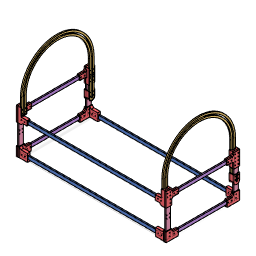
Locolus V2.1 (with correction) v3 (Autodesk Fusion 360 design; units mm, degrees)
Autodesk Fusion 360 part; units mm, degrees
note: some values were not read from the file. Chosen so that the rebuilt part matches the saved one: which bodies a step acts on; which face or edge a step refers to. Set by a fixed rule: which sketch regions a step uses.
sketch "Sketch1" plane through (0, 0, 0) normal (1, 0, 0) x (0, 0, -1) in component "Door"
  line L0 (0, 0) -> (0, 50)
  arc A0 (200, 50) -> (0, 50) centre (100, 50) ccw
  line L1 (200, 50) -> (200, 0)
  line L2 (-5, 0) -> (-5, 50)
  arc A1 (205, 50) -> (-5, 50) centre (100, 50) ccw
  line L3 (205, 50) -> (205, 0)
  line L4 (-9, 0) -> (-9, 50)
  arc A2 (209, 50) -> (-9, 50) centre (100, 50) ccw
  line L5 (209, 50) -> (209, 0)
  line L6 (-14, 0) -> (-14, 50)
  arc A3 (214, 50) -> (-14, 50) centre (100, 50) ccw
  line L7 (214, 50) -> (214, 0)
  line L8 (-5, 0) -> (0, 0)
  line L9 (200, 0) -> (205, 0)
  line L10 (209, 0) -> (214, 0)
  line L11 (-14, 0) -> (-9, 0)
  line L12 (-11.5, 0) -> (-11.5, 50) construction
  line L13 (-2.5, 0) -> (-2.5, 50) construction
  circle A4 centre (-2.5, 5) radius 1.4
  circle A5 centre (-2.5, 15) radius 1.4
  line L14 (-7, 0) -> (-7, 19) construction
  circle A6 centre (-11.5, 5) radius 1.4
  circle A7 centre (-11.5, 15) radius 1.4
  line L15 (100, 50) -> (100, 0) construction
  circle A8 centre (211.5, 15) radius 1.4
  circle A9 centre (211.5, 5) radius 1.4
  circle A10 centre (202.5, 5) radius 1.4
  circle A11 centre (202.5, 15) radius 1.4
  line L16 (200, 0) -> (205, 0)
  line L17 (205, 0) -> (205, -60)
  line L18 (200, -60) -> (200, 0)
  line L19 (209, 0) -> (214, 0)
  line L20 (214, 0) -> (214, -60)
  line L21 (209, -60) -> (209, 0)
  circle A12 centre (202.5, -5) radius 1.4
  circle A13 centre (211.5, -15) radius 1.4
  circle A14 centre (202.5, -15) radius 1.4
  circle A15 centre (211.5, -5) radius 1.4
  line L22 (207, -60) -> (207, -43) construction
  line L23 (211.5, -60) -> (211.5, -39) construction
  line L24 (202.5, -60) -> (202.5, -39) construction
  circle A16 centre (211.5, -55) radius 1.4
  circle A17 centre (211.5, -45) radius 1.4
  circle A18 centre (202.5, -55) radius 1.4
  circle A19 centre (202.5, -45) radius 1.4
  arc A20 (205, -60) -> (209, -60) centre (207, -60) ccw
  arc A21 (200, -60) -> (214, -60) centre (207, -60) ccw
  point P0 (202.5, -45)
  dimension "d1" = 100
  dimension "d2" = 50
  dimension "d3" = -5
  dimension "d4" = -9
  dimension "d5" = -14
  dimension "d6" = 50
  dimension "d7" = 2.8
  dimension "d8" = 5
  dimension "d9" = 2.8
  dimension "d10" = 15
  dimension "d11" = 2
  dimension "d14" = 5
  dimension "d15" = 60
  dimension "d16" = 5
  dimension "d17" = 60
  dimension "d38" = 2
  dimension "d39" = 2.8
  dimension "d40" = 2.8
  dimension "d50" = 5
  dimension "d51" = 9
  dimension "d52" = 15
  constraint coincident L0.start L8.end
  constraint vertical L0
  constraint tangent L0 A0
  constraint tangent A0 L1
  constraint vertical L1
  constraint perpendicular L0 L8
  constraint perpendicular L7 L10
  constraint perpendicular L4 L11
  constraint midpoint L11 L12.start
  constraint perpendicular L11 L12
  constraint midpoint L8 L13.start
  constraint perpendicular L8 L13
  constraint coincident L13 A4.centre
  constraint coincident L13 A5.centre
  constraint parallel L2 L14
  constraint symmetric A4 L14 A6
  constraint symmetric A5 L14 A7
  constraint coincident A0.centre A1.centre
  constraint vertical L15
  constraint symmetric A4 L15 A10
  constraint symmetric A5 L15 A11
  constraint symmetric A6 L15 A9
  constraint symmetric A7 L15 A8
  constraint horizontal L16
  constraint vertical L17
  constraint vertical L18
  constraint horizontal L19
  constraint vertical L20
  constraint vertical L21
  constraint symmetric L9 A8 A13
  constraint symmetric L9 A9 A15
  constraint symmetric L9 A10 A12
  constraint symmetric L9 A11 A14
  constraint coincident L23 A16.centre
  constraint coincident L23 A17.centre
  constraint symmetric L22 A16 A18
  constraint symmetric L22 A17.centre P0
  constraint symmetric L22 A17 A19
  constraint tangent L17 A20
  constraint tangent L21 A20
  constraint tangent L18 A21
  constraint tangent L20 A21
  constraint vertical L23
  constraint vertical L24
  measures "d1" radius of A0
  measures "d2" distance of L0.start L0.end
  measures "d6" distance of A0.start L1.end
  measures "d7" diameter of A4
  measures "d8" distance of L8 A4.centre
  measures "d9" diameter of A5
  measures "d10" distance of L8 A5.centre
  measures "d11" distance of L4 L14
  measures "d14" distance of L1.end L3.end
  measures "d15" distance of L1.end L18.start
  measures "d16" distance of L5.end L7.end
  measures "d17" distance of L5.end L21.start
  measures "d38" distance of L17 L22
  measures "d39" diameter of A16
  measures "d40" diameter of A17
  measures "d50" vertical distance of A18.centre L22.start
  measures "d51" distance of A16.centre A18.centre
  measures "d52" vertical distance of P0 L22.start
extrude "Extrude1" add sketch "Sketch1" against normal blind 4 contours L0 A0 L1 L2 A1 L3 L8 L9 L16 | L4 A2 L5 L6 A3 L7 L10 L11 L19 makes body 1 at (0, 38.8, 11.5) makes body 2 at (0, 38.798, 2.4569) in component "Door"
extrude "Extrude2" add sketch "Sketch1" against normal blind 4 separate body contours L9 L10 L16 L17 L18 L19 L20 L21 A20 A21 makes body 3 in component "Door"
sketch "Sketch1 (2)" plane through (0, 0, 0) normal (1, 0, 0) x (0, 0, -1) in component "Transverse carcas"
  line L0 (195, 0) -> (5, 0)
  line L1 (5, 0) -> (5, 10)
  line L2 (5, 10) -> (195, 10)
  line L3 (195, 10) -> (195, 0)
  line L4 (200, 50) -> (200, 0)
  line L5 (0, 0) -> (0, 50)
  circle A0 centre (190, 5) radius 1.4
  circle A1 centre (180, 5) radius 1.4
  line L6 (100, 10) -> (100, 0) construction
  line L7 (100, 50) -> (100, 0) construction
  circle A2 centre (20, 5) radius 1.4
  circle A3 centre (10, 5) radius 1.4
  circle A4 centre (190, 5) radius 5
  circle A5 centre (10, 5) radius 5
  line L8 (195, -110) -> (5, -110)
  line L9 (5, -110) -> (5, -100)
  line L10 (5, -100) -> (195, -100)
  line L11 (195, -100) -> (195, -110)
  line L12 (200, -60) -> (200, 0)
  line L13 (195, -50) -> (5, -50) construction
  circle A6 centre (190, -105) radius 1.4
  circle A7 centre (190, -105) radius 5
  circle A8 centre (180, -105) radius 1.4
  circle A9 centre (20, -105) radius 1.4
  circle A10 centre (10, -105) radius 5
  circle A11 centre (10, -105) radius 1.4
  point P0 (100, 50)
  dimension "d20" = 5
  dimension "d21" = 5
  dimension "d22" = 10
  dimension "d23" = 40
  dimension "d24" = 2.8
  dimension "d25" = 5
  dimension "d26" = 2.8
  dimension "d27" = 15
  dimension "d28" = 5
  dimension "d29" = 5
  dimension "d30" = 100
  dimension "d31" = 10
  dimension "d32" = 5
  dimension "d33" = 5
  dimension "d34" = 50
  constraint horizontal L0
  constraint vertical L1
  constraint horizontal L2
  constraint vertical L3
  constraint midpoint L2 L6.start
  constraint midpoint L0 L6.end
  constraint symmetric A0 L7 A3
  constraint symmetric A1 L7 A2
  constraint concentric A0 A4
  constraint tangent L0 A4
  constraint concentric A3 A5
  constraint tangent L0 A5
  constraint horizontal L8
  constraint vertical L9
  constraint horizontal L10
  constraint vertical L11
  constraint parallel L0 L13
  constraint symmetric A0 L13 A6
  constraint symmetric A1 L13 A8
  constraint symmetric A2 L13 A9
  constraint symmetric A3 L13 A11
  constraint symmetric A4 L13 A7
  constraint symmetric A5 L13 A10
  measures "d20" distance of L3 L4
  measures "d21" distance of L1 L5
  measures "d22" distance of L0.start L2.end
  measures "d23" distance of L2 P0
  measures "d24" diameter of A0
  measures "d25" distance of L3 A0.centre
  measures "d26" diameter of A1
  measures "d27" distance of L3 A1.centre
  measures "d28" distance of L2 A0.centre
  measures "d29" distance of L2 A1.centre
  measures "d30" distance of L0 L10
  measures "d31" distance of L8 L10
  measures "d32" distance of L11 L12
  measures "d33" distance of L5 L9
  measures "d34" distance of L0 L13
extrude "Extrude1'" add sketch "Sketch1 (2)" against normal blind 4 from surface at -9 separate body contours L0 L2 A4 A5 | A4 | A5 | L8 L10 A7 A10 | A7 | A10 makes body 4 at (-9, 1.2159, -73.4541) makes body 5 at (-9, -108.7841, -73.4541) in component "Transverse carcas"
sketch "Sketch1 (3)" plane through (0, 0, 0) normal (1, 0, 0) x (0, 0, -1) in component "High carcas"
  line L0 (214, 20) -> (200, 20)
  line L1 (200, 20) -> (200, -110)
  line L2 (200, -110) -> (214, -110)
  line L3 (214, -110) -> (214, 20)
  line L4 (214, 0) -> (214, -60)
  line L5 (200, -60) -> (200, 0)
  line L6 (190, -110) -> (10, -110)
  circle A0 centre (211.5, 15) radius 1.4
  circle A1 centre (202.5, 15) radius 1.4
  circle A2 centre (211.5, -15) radius 1.4
  circle A3 centre (211.5, -5) radius 1.4
  circle A4 centre (211.5, 5) radius 1.4
  circle A5 centre (202.5, 5) radius 1.4
  circle A6 centre (202.5, -5) radius 1.4
  circle A7 centre (202.5, -15) radius 1.4
  circle A8 centre (202.5, -55) radius 1.4
  line L7 (202.5, -60) -> (202.5, -39)
  circle A9 centre (202.5, -45) radius 1.4
  circle A10 centre (211.5, -55) radius 1.4
  circle A11 centre (211.5, -45) radius 1.4
  line L8 (214, 50) -> (214, 0)
  line L9 (100, 50) -> (100, 0)
  circle A12 centre (-11.5, 15) radius 1.4
  circle A13 centre (-2.5, -55) radius 1.4
  line L10 (0, -60) -> (0, 0)
  line L11 (0, -110) -> (-14, -110)
  circle A14 centre (-11.5, -45) radius 1.4
  circle A15 centre (-11.5, -55) radius 1.4
  circle A16 centre (-2.5, -45) radius 1.4
  line L12 (-2.5, -60) -> (-2.5, -39)
  line L13 (-14, -110) -> (-14, 20)
  line L14 (0, 20) -> (0, -110)
  line L15 (-14, 0) -> (-14, -60)
  circle A17 centre (-11.5, 5) radius 1.4
  circle A18 centre (-2.5, 15) radius 1.4
  circle A19 centre (-2.5, 5) radius 1.4
  circle A20 centre (-2.5, -15) radius 1.4
  circle A21 centre (-2.5, -5) radius 1.4
  line L16 (-14, 20) -> (0, 20)
  line L17 (214, -110) -> (235.1047, -110) construction
  line L18 (205, -110) -> (205, -95) construction
  circle A22 centre (205, -105) radius 1.4
  circle A23 centre (205, -95) radius 1.4
  circle A24 centre (-5, -105) radius 1.4
  circle A25 centre (-5, -95) radius 1.4
  line L19 (-5, -110) -> (-5, -95) construction
  point P0 (211.5, 15)
  point P1 (211.5, -15)
  point P2 (-11.5, -15)
  point P3 (-14, 0)
  point P4 (-11.5, 15)
  dimension "d44" = 5
  dimension "d104" = 5
  dimension "d105" = 2.8
  dimension "d106" = 2.8
  dimension "d107" = 5
  dimension "d108" = 15
  constraint horizontal L0
  constraint vertical L1
  constraint horizontal L2
  constraint vertical L3
  constraint collinear L3 L4
  constraint collinear L1 L5
  constraint collinear L2 L6
  constraint symmetric L0.start L9 L13.end
  constraint symmetric L0.end L9 L14.start
  constraint symmetric L1.end L9 L11.start
  constraint symmetric L2.end L9 L11.end
  constraint symmetric L4.start L9 P3
  constraint symmetric L4.end L9 L15.end
  constraint symmetric L5.start L9 L10.start
  constraint symmetric L5.end L9 L10.end
  constraint symmetric P0 L9 P4
  constraint symmetric A0 L9 A12
  constraint symmetric A1 L9 A18
  constraint symmetric P1 L9 P2
  constraint symmetric A4 L9 A17
  constraint symmetric A5 L9 A19
  constraint symmetric A6 L9 A21
  constraint symmetric A7 L9 A20
  constraint symmetric A8 L9 A13
  constraint symmetric L7.start L9 L12.start
  constraint symmetric L7.end L9 L12.end
  constraint symmetric A9 L9 A16
  constraint symmetric A10 L9 A15
  constraint symmetric A11 L9 A14
  constraint horizontal L17
  constraint coincident L2 L18.start
  constraint perpendicular L2 L18
  constraint coincident L18 A22.centre
  constraint coincident L18 A23.centre
  constraint symmetric L9 L18.start L19.start
  constraint symmetric L9 L18.end A25.centre
  constraint symmetric L9 A22 A24
  constraint symmetric L9 A23 A25
  measures "d44" distance of L0 P0
  measures "d104" distance of L1 L18
  measures "d105" diameter of A22
  measures "d106" diameter of A23
  measures "d107" distance of L2 A22.centre
  measures "d108" distance of L2 L18.end
extrude "Extrude1''" add sketch "Sketch1 (3)" along normal blind 4 from surface at -13 separate body makes body 6 at (-13, -18.4191, 9.6485) makes body 7 at (-13, -68.7664, -206.3764) in component "High carcas"
ref_plane "WorkPlane1" through (-11, -45, -211) normal (0, 0, -1) x (0, 1, 0) in component "Along carcas"
sketch "Sketch1 (4)" plane through (-11, -48.5, -211) normal (0, 0, -1) x (1, 0, 0) in component "Along carcas"
  line L0 (2, 61.5) -> (2, -68.5)
  line L1 (7, 61.5) -> (7, 51.5)
  line L2 (7, 51.5) -> (457, 51.5)
  line L3 (7, 61.5) -> (457, 61.5)
  line L4 (457, 61.5) -> (457, 51.5)
  line L5 (7, 56.5) -> (52.3362, 56.5) construction
  line L6 (232, 51.5) -> (232, 61.5) construction
  circle A0 centre (12, 56.5) radius 1.4
  circle A1 centre (22, 56.5) radius 1.4
  circle A2 centre (442, 56.5) radius 1.4
  circle A3 centre (452, 56.5) radius 1.4
  circle A4 centre (12, 56.5) radius 5
  circle A5 centre (452, 56.5) radius 5
  point P0 (2, 51.5)
  dimension "d61" = 450
  dimension "d62" = 5
  dimension "d64" = 10
  dimension "d65" = 450
  dimension "d66" = 10
  dimension "d67" = 2.8
  dimension "d68" = 2.8
  dimension "d69" = 5
  dimension "d70" = 15
  constraint parallel L0 L1
  constraint perpendicular L0 L2
  constraint perpendicular L1 L3
  constraint midpoint L1 L5.start
  constraint perpendicular L1 L5
  constraint midpoint L2 L6.start
  constraint midpoint L3 L6.end
  constraint coincident L5 A0.centre
  constraint coincident L5 A1.centre
  constraint symmetric L6 A0 A3
  constraint symmetric L6 A1 A2
  constraint concentric A0 A4
  constraint tangent L3 A4
  constraint concentric A3 A5
  constraint tangent L3 A5
  measures "d61" distance of L1.end L2.end
  measures "d62" distance of L0 L1
  measures "d64" distance of L0.start L2
  measures "d65" distance of L1.start L3.end
  measures "d66" distance of L2.end L3.end
  measures "d67" diameter of A0
  measures "d68" diameter of A1
  measures "d69" distance of L1 A0.centre
  measures "d70" distance of L1 A1.centre
extrude "Extrude1'''" add sketch "Sketch1 (4)" along normal mid plane 4 separate body contours A4 | L2 L3 A4 A5 | A5 makes body 8 in component "Along carcas"
sketch "Sketch1 (5)" plane through (-13, 0, 0) normal (-1, 0, 0) x (0, 0, 1) in component "Connections"
  line L0 (-214, 20) -> (-214, -110)
  line L1 (-214, -110) -> (-200, -110)
  line L2 (-200, -110) -> (-200, 20)
  circle A0 centre (-211.5, 5) radius 1.4
  circle A1 centre (-202.5, -45) radius 1.4
  circle A2 centre (-202.5, -55) radius 1.4
  circle A3 centre (-211.5, 15) radius 1.4
  circle A4 centre (-211.5, -15) radius 1.4
  circle A5 centre (-202.5, 15) radius 1.4
  circle A6 centre (-211.5, -55) radius 1.4
  circle A7 centre (-211.5, -45) radius 1.4
  circle A8 centre (-202.5, -5) radius 1.4
  circle A9 centre (-202.5, -15) radius 1.4
  circle A10 centre (-202.5, 5) radius 1.4
  circle A11 centre (-211.5, -5) radius 1.4
  circle A12 centre (-180, -105) radius 1.4
  circle A13 centre (-10, -105) radius 1.4
  circle A14 centre (-20, -105) radius 1.4
  circle A15 centre (-190, -105) radius 1.4
  arc A16 (-190, -100) -> (-190, -110) centre (-190, -105) ccw
  line L3 (-190, -110) -> (-10, -110)
  arc A17 (-10, -110) -> (-10, -100) centre (-10, -105) ccw
  line L4 (-10, -100) -> (-190, -100)
  line L5 (-213, -106.4) -> (-213, -103.6)
  line L6 (-213, -106.4) -> (-213, -103.6)
  line L7 (-213, -106.4) -> (-213, -103.6)
  line L8 (-213, -106.4) -> (-213, -103.6)
  line L9 (-213, -100) -> (-213, -110)
  line L10 (-213, -100) -> (-213, -110)
  line L11 (-209, -110) -> (-209, -100)
  line L12 (-213, -100) -> (-213, -110)
  line L13 (-177, -99.9) -> (-177, -97.9)
  line L14 (-177, -97.9) -> (-197.9, -97.9)
  line L15 (-197.9, -97.9) -> (-197.9, -87.9)
  line L16 (-197.9, -87.9) -> (-199.9, -87.9)
  line L17 (-199.9, -87.9) -> (-199.9, -110.1)
  line L18 (-177, -99.9) -> (-195.1, -99.9)
  line L19 (-195.1, -99.9) -> (-195.1, -110.1)
  line L20 (-195.1, -110.1) -> (-177, -110.1)
  line L21 (-177, -110.1) -> (-177, -117.1)
  line L22 (-177, -117.1) -> (-216.1, -117.1)
  line L23 (-216.1, -117.1) -> (-216.1, -87.9)
  line L24 (-216.1, -87.9) -> (-214.1, -87.9)
  line L25 (-214.1, -87.9) -> (-214.1, -110.1)
  line L26 (-214.1, -110.1) -> (-199.9, -110.1)
  line L27 (-180, -105) -> (-190, -105) construction
  line L28 (-214.1, -87.9) -> (-199.9, -87.9)
  line L29 (-177, -99.9) -> (-177, -110.1)
  line L30 (-197.9, -92.2431) -> (-192.2431, -97.9)
  line L31 (-197.9, -92.2431) -> (-191.0674, -92.2431) construction
  circle A18 centre (-205, -105) radius 1.4
  circle A19 centre (-205, -95) radius 1.4
  line L32 (-200, 20) -> (-214, 20)
  dimension "d73" = 2
  dimension "d74" = 0.1
  dimension "d75" = 10
  dimension "d76" = 0.1
  dimension "d77" = 0.1
  dimension "d78" = 2
  dimension "d79" = 0.1
  dimension "d80" = 2
  dimension "d82" = 3
  dimension "d83" = 0.1
  dimension "d84" = 7
  dimension "d85" = 5.1
  dimension "d88" = 45
  dimension "d89" = 8
  constraint parallel L2 L13
  constraint perpendicular L0 L14
  constraint perpendicular L14 L15
  constraint perpendicular L15 L16
  constraint perpendicular L14 L17
  constraint perpendicular L2 L18
  constraint perpendicular L18 L19
  constraint perpendicular L19 L20
  constraint perpendicular L20 L21
  constraint perpendicular L21 L22
  constraint perpendicular L22 L23
  constraint perpendicular L23 L24
  constraint perpendicular L24 L25
  constraint perpendicular L25 L26
  constraint coincident A12.centre L27.start
  constraint coincident A15.centre A16.centre
  constraint collinear L13 L21
  constraint collinear L16 L24
  constraint horizontal L31
  constraint coincident L15 L30.start
  constraint coincident L14 L30.end
  measures "d73" distance of L15 L17
  measures "d74" distance of L2 L17
  measures "d75" distance of L14.end L15.end
  measures "d76" distance of L1 L26
  measures "d77" distance of L0 L25
  measures "d78" distance of L23 L25
  measures "d79" distance of L4 L18
  measures "d80" distance of L14 L18
  measures "d82" distance of A12.centre L13
  measures "d83" distance of L3 L20
  measures "d84" distance of L20 L22
  measures "d85" distance of A15.centre L19
  measures "d88" angle of L30 L31
  measures "d89" distance of L30.start L30.end
extrude "Extrude1''''" add sketch "Sketch1 (5)" along normal blind 2 separate body contours L0 L1 L2 L28 | L0 L1 L2 L17 L25 L26 L28 | L13 L14 L15 L16 L17 L18 L19 L20 L21 L22 L23 L24 L25 L26 | L14 L15 L30 | A16 L3 L4 L18 L19 L20 L29 | A16 L3 L4 L29 makes body 9 in component "Connections"
extrude "Extrude2'" add sketch "Sketch1 (5)" against normal blind 2 contours L13 L14 L15 L16 L17 L18 L19 L20 L21 L22 L23 L24 L25 L26 | L14 L15 L30 bodies 9 in component "Connections"
extrude "Extrude3" add sketch "Sketch1 (5)" against normal blind 2 from surface at -4 separate body contours L0 L1 L2 L28 | L0 L1 L2 L17 L25 L26 L28 | L13 L14 L15 L16 L17 L18 L19 L20 L21 L22 L23 L24 L25 L26 | L14 L15 L30 | A16 L3 L4 L18 L19 L20 L29 | A16 L3 L4 L29 makes body 10 in component "Connections"
extrude "Extrude4" add sketch "Sketch1 (5)" along normal blind 2 from surface at -4 contours L13 L14 L15 L16 L17 L18 L19 L20 L21 L22 L23 L24 L25 L26 | L14 L15 L30 bodies 10 in component "Connections"
sketch "Sketch2" plane through (0, 0, -213) normal (0, 0, -1) x (-1, 0, 0) in component "Connections"
  circle A0 centre (-431, -105) radius 1.4
  circle A1 centre (-11, -105) radius 1.4
  circle A2 centre (-1, -105) radius 1.4
  circle A3 centre (-441, -105) radius 1.4
  arc A4 (-1, -110) -> (-1, -100) centre (-1, -105) ccw
  line L0 (-1, -100) -> (-441, -100)
  arc A5 (-441, -100) -> (-441, -110) centre (-441, -105) ccw
  line L1 (-441, -110) -> (-1, -110)
  line L2 (7, -117.1) -> (7, -87.9)
  line L3 (-19, -110.1) -> (4.1, -110.1)
  line L4 (4.1, -110.1) -> (4.1, -99.9)
  line L5 (4.1, -99.9) -> (-19, -99.9)
  line L6 (-19, -99.9) -> (-19, -92.9)
  line L7 (-19, -92.9) -> (7, -92.9)
  line L8 (-19, -110.1) -> (-19, -117.1)
  line L9 (-19, -117.1) -> (7, -117.1)
  line L10 (-19, -99.9) -> (-19, -110.1)
  line L11 (7, -87.9) -> (2, -92.9)
  dimension "d98" = 0.1
  dimension "d99" = 5.1
  dimension "d100" = 0.1
  dimension "d101" = 8
  dimension "d102" = 45
  dimension "d103" = 7
  constraint perpendicular L3 L4
  constraint parallel L0 L5
  constraint perpendicular L5 L6
  constraint coincident L2 L7.end
  constraint perpendicular L2 L7
  constraint perpendicular L3 L8
  constraint coincident L2.start L9.end
  constraint perpendicular L4 L5
  constraint collinear L6 L8
  constraint perpendicular L8 L9
  constraint coincident L2.end L11.start
  constraint coincident L7 L11.end
  measures "d98" distance of L1 L3
  measures "d99" distance of A2.centre L4
  measures "d100" distance of L0 L5
  measures "d101" distance of A1.centre L8
  measures "d102" angle of L7 L11
  measures "d103" distance of L5.end L6.end
extrude "Extrude5" add sketch "Sketch2" along normal blind 2 contours A4 L0 L1 L10 | A4 L0 L1 L3 L4 L5 L10 | L2 L3 L4 L5 L6 L7 L8 L9 | L2 L7 L11 bodies 10 in component "Connections"
extrude "Extrude6" add sketch "Sketch2" against normal blind 4 contours L2 L3 L4 L5 L6 L7 L8 L9 | L2 L7 L11 bodies 10 in component "Connections"
extrude "Extrude7" add sketch "Sketch2" against normal blind 2 from surface at -4 contours A4 L0 L1 L10 | A4 L0 L1 L3 L4 L5 L10 | L2 L3 L4 L5 L6 L7 L8 L9 | L2 L7 L11 bodies 10 in component "Connections"
ref_plane "WorkPlane1" through (-11, -45, -100) normal (0, 0, 1) x (0, -1, 0) in component "Carcas"
mirror "Mirror1" about plane through (-11, -45, -100) normal (0, 0, 1) of bodies 9 10 makes body 11 at (-15, -113.5216, -5.5295) makes body 12 at (-7, -113.532, -8.6318) in component "Connections"
mirror "Mirror1'" about plane through (-11, -45, -100) normal (0, 0, 1) of bodies 8 makes body 13 in component "Along carcas"
ref_plane "WorkPlane2" through (221, -45, 7) normal (1, 0, 0) x (0, 0, -1) in component "Carcas"
mirror "Mirror2" about plane through (221, -45, 7) normal (1, 0, 0) of bodies 11 12 10 9 makes body 14 at (457, -113.5216, -194.4705) makes body 15 at (449, -113.532, -191.3682) makes body 16 at (457, -113.5216, -5.5295) makes body 17 at (449, -113.532, -8.6318) in component "Connections"
mirror "Mirror1''" about plane through (221, -45, 7) normal (1, 0, 0) of bodies 5 4 makes body 18 at (451, 1.2159, -73.4541) makes body 19 at (451, -108.7841, -73.4541) in component "Transverse carcas"
mirror "Mirror1'''" about plane through (221, -45, 7) normal (1, 0, 0) of bodies 6 7 makes body 20 at (455, -18.4191, 9.6485) makes body 21 at (455, -68.7664, -206.3764) in component "High carcas"
mirror "Mirror1''''" about plane through (221, -45, 7) normal (1, 0, 0) of bodies 2 1 3 makes body 22 at (442, 38.8, 11.5) makes body 23 at (442, 38.798, 2.4569) makes body 24 at (442, -1.2013, -211.4651) in component "Door"
copy_body "CopyPasteBodies1" bodies 8 13 makes body 25 makes body 26 in component "Along carcas"
move_body "Move1" bodies 25 26 to x (1, 0, 0) y (0, 1, 0) z (0, 0, 1) at (0, 95, 0) in component "Along carcas"
sketch "Sketch3" plane through (-13, 0, 0) normal (-1, 0, 0) x (0, 0, 1) in component "Connections"
  line L0 (-200, 20) -> (-214, 20)
  line L1 (-214, 20) -> (-214, -110)
  line L2 (-214, -110) -> (-200, -110)
  line L3 (-200, -110) -> (-200, 20)
  circle A0 centre (-211.5, 15) radius 1.4
  circle A1 centre (-211.5, -45) radius 1.4
  circle A2 centre (-211.5, -55) radius 1.4
  circle A3 centre (-202.5, -45) radius 1.4
  circle A4 centre (-211.5, 5) radius 1.4
  circle A5 centre (-211.5, -15) radius 1.4
  circle A6 centre (-202.5, -55) radius 1.4
  circle A7 centre (-202.5, -15) radius 1.4
  circle A8 centre (-202.5, -5) radius 1.4
  circle A9 centre (-202.5, 5) radius 1.4
  circle A10 centre (-202.5, 15) radius 1.4
  circle A11 centre (-211.5, -5) radius 1.4
  circle A12 centre (-205, -95) radius 1.4
  circle A13 centre (-205, -105) radius 1.4
  circle A14 centre (-202.5, -45) radius 1.4
  circle A15 centre (-211.5, -55) radius 1.4
  circle A16 centre (-211.5, -45) radius 1.4
  circle A17 centre (-202.5, -55) radius 1.4
  line L4 (-200, -60) -> (-200, 0)
  line L5 (-200, 0) -> (-205, 0)
  line L6 (-205, 0) -> (-205, -60)
  arc A18 (-209, -60) -> (-205, -60) centre (-207, -60) ccw
  line L7 (-209, -60) -> (-209, 0)
  line L8 (-209, 0) -> (-214, 0)
  line L9 (-214, 0) -> (-214, -60)
  arc A19 (-214, -60) -> (-200, -60) centre (-207, -60) ccw
  line L10 (-198, -60) -> (-198, 2)
  line L11 (-198, 2) -> (-207, 2)
  line L12 (-207, 2) -> (-216, 2)
  line L13 (-216, 2) -> (-216, -60)
  arc A20 (-216, -60) -> (-198, -60) centre (-207, -60) ccw
  line L14 (-216, -40) -> (-209, -40)
  line L15 (-205, -40) -> (-198, -40)
  circle A21 centre (-202.5, -15) radius 1.4
  circle A22 centre (-211.5, -5) radius 1.4
  circle A23 centre (-202.5, -5) radius 1.4
  circle A24 centre (-211.5, -15) radius 1.4
  dimension "d130" = 5
  dimension "d131" = 2
  constraint perpendicular L7 L14
  constraint horizontal L14
  constraint coincident L13 L14.start
  constraint coincident L10 L15.end
  constraint coincident L7 L14.end
  constraint coincident L6 L15.start
  constraint collinear L14 L15
  measures "d130" distance of A1.centre L14
extrude "Extrude9" add sketch "Sketch3" along normal blind -13 and the other way blind -2 separate body contours L3 L4 L10 A20 L15 | L1 L9 L13 A20 L14 makes body 27 at (-5, -48.5523, -214) makes body 28 at (-10, -57.1046, -200) in component "Connections"
extrude "Extrude10" add sketch "Sketch3" against normal blind 9 from surface at -4 contours L1 L3 A19 A20 bodies 27 28 in component "Connections"
extrude "Extrude11" add sketch "Sketch3" along normal blind 2 contours L1 L3 L4 L6 A18 L7 L9 A19 L14 L15 | L1 L3 A19 A20 bodies 27 in component "Connections"
mirror "Mirror3" about plane through (221, -45, 7) normal (1, 0, 0) of bodies 27 makes body 29 in component "Connections"
sketch "Sketch4" plane through (-13, 0, 0) normal (-1, 0, 0) x (0, 0, 1) in component "Connections"
  circle A0 centre (-10, 5) radius 1.4
  circle A1 centre (-190, 5) radius 1.4
  circle A2 centre (-20, 5) radius 1.4
  circle A3 centre (-180, 5) radius 1.4
  arc A4 (-190, 10) -> (-190, 0) centre (-190, 5) ccw
  line L0 (-190, 0) -> (-10, 0)
  arc A5 (-10, 0) -> (-10, 10) centre (-10, 5) ccw
  line L1 (-10, 10) -> (-190, 10)
  line L2 (-200, 20) -> (-214, 20)
  line L3 (-214, 20) -> (-214, -110)
  line L4 (-214, -110) -> (-200, -110)
  line L5 (-200, -110) -> (-200, 20)
  circle A6 centre (-211.5, 15) radius 1.4
  circle A7 centre (-211.5, -45) radius 1.4
  circle A8 centre (-211.5, -55) radius 1.4
  circle A9 centre (-202.5, -45) radius 1.4
  circle A10 centre (-211.5, 5) radius 1.4
  circle A11 centre (-211.5, -15) radius 1.4
  circle A12 centre (-202.5, -55) radius 1.4
  circle A13 centre (-202.5, -15) radius 1.4
  circle A14 centre (-202.5, -5) radius 1.4
  circle A15 centre (-202.5, 5) radius 1.4
  circle A16 centre (-202.5, 15) radius 1.4
  circle A17 centre (-211.5, -5) radius 1.4
  circle A18 centre (-205, -95) radius 1.4
  circle A19 centre (-205, -105) radius 1.4
  line L6 (-214.1, 20.1) -> (-214.1, -110.1)
  line L7 (-214.1, -110.1) -> (-199.9, -110.1)
  line L8 (-199.9, -110.1) -> (-199.9, 20.1)
  line L9 (-199.9, 20.1) -> (-214.1, 20.1)
  line L10 (-176, 10.1) -> (-176, -0.1)
  line L11 (-176, -0.1) -> (-195.1, -0.1)
  line L12 (-195.1, -0.1) -> (-195.1, 10.1)
  line L13 (-195.1, 10.1) -> (-176, 10.1)
  line L14 (-176, 10.1) -> (-176, 12.1)
  line L15 (-176, 12.1) -> (-199.9, 12.1)
  line L16 (-199.9, 20.1) -> (-197.9, 20.1)
  line L17 (-197.9, 20.1) -> (-197.9, 12.1)
  line L18 (-180, 5) -> (-190, 5) construction
  line L19 (-176, -2.1) -> (-199.9, -2.1)
  line L20 (-176, -0.1) -> (-176, -2.1)
  line L21 (-197.9, 16.1) -> (-193.9, 12.1)
  line L22 (-197.9, 16.1) -> (-191.395, 16.1) construction
  line L23 (-216.1, -23) -> (-216.1, 20.1)
  line L24 (-216.1, 20.1) -> (-214.1, 20.1)
  line L25 (-216.1, 20.1) -> (-216.1, 23)
  line L26 (-216.1, 23) -> (-197.9, 23)
  line L27 (-197.9, 20.1) -> (-197.9, 23)
  line L28 (-197.9, -2.1) -> (-197.9, -23)
  line L29 (-197.9, -23) -> (-216.1, -23)
  line L30 (-197.9, -6.1) -> (-193.9, -2.1)
  dimension "d146" = 0.1
  dimension "d147" = 0.1
  dimension "d148" = 5.1
  dimension "d149" = 0.1
  dimension "d150" = 4
  dimension "d151" = 2
  dimension "d152" = 2
  dimension "d155" = 45
  dimension "d160" = 8
  dimension "d161" = 8
  dimension "d162" = 2
  dimension "d163" = 2
  constraint perpendicular L0 L10
  constraint perpendicular L10 L11
  constraint perpendicular L11 L12
  constraint horizontal L13
  constraint perpendicular L13 L14
  constraint coincident L8 L15.end
  constraint perpendicular L8 L15
  constraint perpendicular L8 L16
  constraint perpendicular L16 L17
  constraint coincident A3.centre L18.start
  constraint coincident A1.centre A4.centre
  constraint symmetric L10.start L18 L10.end
  constraint symmetric L14.end L18 L19.start
  constraint symmetric L15.end L18 L19.end
  constraint coincident L15 L17.end
  constraint horizontal L22
  constraint midpoint L17 L21.start
  constraint coincident L15 L21.end
  constraint perpendicular L23 L24
  constraint perpendicular L24 L25
  constraint perpendicular L23 L26
  constraint perpendicular L16 L27
  constraint coincident L19 L28.start
  constraint perpendicular L19 L28
  constraint perpendicular L3 L29
  constraint perpendicular L26 L27
  constraint symmetric L18 L21.start L30.start
  constraint symmetric L18 L21.end L30.end
  measures "d147" distance of L1 L13
  measures "d148" distance of A1.centre L12
  measures "d149" distance of L0 L11
  measures "d150" distance of A3.centre L10
  measures "d151" distance of L10.start L14.end
  measures "d152" distance of L8.end L16.end
  measures "d155" angle of L21 L22
  measures "d160" distance of A11.centre L29
  measures "d161" distance of A6.centre L26
  measures "d162" distance of L8 L28
  measures "d163" distance of L6 L23
extrude "Extrude12" add sketch "Sketch4" along normal blind 2 separate body contours A4 L0 L1 L10 | A4 L0 L1 L10 L11 L12 L13 | L8 L11 L12 L13 L14 L15 L19 L20 | L15 L17 L21 | L19 L28 L30 | L8 L15 L16 L17 | L8 L19 L28 L29 | L2 L3 L5 L6 L8 L9 L29 | L9 L16 L24 L25 L26 L27 | L6 L23 L24 L29 | L2 L3 L5 L29 makes body 30 in component "Connections"
extrude "Extrude13" add sketch "Sketch4" against normal blind 2 contours L8 L11 L12 L13 L14 L15 L19 L20 | L15 L17 L21 | L19 L28 L30 | L8 L15 L16 L17 | L8 L19 L28 L29 | L9 L16 L24 L25 L26 L27 | L6 L23 L24 L29 bodies 30 in component "Connections"
extrude "Extrude14" add sketch "Sketch4" along normal blind 2 from surface at -4 separate body contours L8 L11 L12 L13 L14 L15 L19 L20 | L15 L17 L21 | L19 L28 L30 | L8 L15 L16 L17 | L8 L19 L28 L29 | L9 L16 L24 L25 L26 L27 | L6 L23 L24 L29 makes body 31 in component "Connections"
extrude "Extrude15" add sketch "Sketch4" against normal blind 2 from surface at -4 contours A4 L0 L1 L10 | A4 L0 L1 L10 L11 L12 L13 | L8 L11 L12 L13 L14 L15 L19 L20 | L15 L17 L21 | L19 L28 L30 | L8 L15 L16 L17 | L8 L19 L28 L29 | L2 L3 L5 L6 L8 L9 L29 | L9 L16 L24 L25 L26 L27 | L6 L23 L24 L29 | L2 L3 L5 L29 bodies 31 in component "Connections"
sketch "Sketch5" plane through (-7, 0, 0) normal (1, 0, 0) x (0, 0, -1) in component "Connections"
  line L0 (193.9, -2.1) -> (197.9, -6.1)
  line L1 (197.9, -6.1) -> (197.9, -23)
  line L2 (197.9, -23) -> (216.1, -23)
  line L3 (216.1, -23) -> (216.1, 23)
  line L4 (216.1, 23) -> (197.9, 23)
  line L5 (197.9, 23) -> (197.9, 16.1)
  line L6 (197.9, 16.1) -> (193.9, 12.1)
  line L7 (193.9, 12.1) -> (176, 12.1)
  line L8 (176, 12.1) -> (176, -2.1)
  line L9 (176, -2.1) -> (193.9, -2.1)
  circle A0 centre (202.5, -5) radius 1.4
  circle A1 centre (202.5, 5) radius 1.4
  circle A2 centre (190, 5) radius 1.4
  circle A3 centre (180, 5) radius 1.4
  circle A4 centre (211.5, -5) radius 1.4
  circle A5 centre (211.5, -15) radius 1.4
  circle A6 centre (202.5, 15) radius 1.4
  circle A7 centre (211.5, 5) radius 1.4
  circle A8 centre (202.5, -15) radius 1.4
  circle A9 centre (211.5, 15) radius 1.4
  circle A10 centre (202.5, -55) radius 1.4
  circle A11 centre (211.5, -45) radius 1.4
  circle A12 centre (202.5, -15) radius 1.4
  circle A13 centre (211.5, -5) radius 1.4
  circle A14 centre (202.5, -5) radius 1.4
  circle A15 centre (211.5, -15) radius 1.4
  circle A16 centre (211.5, -55) radius 1.4
  circle A17 centre (202.5, -45) radius 1.4
  line L10 (200, 0) -> (200, -60)
  arc A18 (200, -60) -> (214, -60) centre (207, -60) ccw
  line L11 (214, -60) -> (214, 0)
  line L12 (214, 0) -> (209, 0)
  line L13 (209, 0) -> (209, -60)
  arc A19 (205, -60) -> (209, -60) centre (207, -60) ccw
  line L14 (205, -60) -> (205, 0)
  line L15 (205, 0) -> (200, 0)
  circle A20 centre (211.5, 5) radius 1.4
  circle A21 centre (211.5, 5) radius 1.4
  circle A22 centre (-11.5, 15) radius 1.4
  circle A23 centre (211.5, 15) radius 1.4
  circle A24 centre (-11.5, 5) radius 1.4
  arc A25 (214, 50) -> (-14, 50) centre (100, 50) ccw
  line L16 (-14, 50) -> (-14, 0)
  line L17 (-14, 0) -> (-9, 0)
  line L18 (-9, 0) -> (-9, 50)
  arc A26 (209, 50) -> (-9, 50) centre (100, 50) ccw
  line L19 (209, 50) -> (209, 0)
  line L20 (209, 0) -> (214, 0)
  line L21 (214, 0) -> (214, 50)
  line L22 (211.5, -23) -> (211.5, 23)
  line L23 (207, -23) -> (207, 23) construction
  line L24 (202.5, -23) -> (202.5, 23)
  line L25 (197.9, 16.1) -> (197.9, -6.1)
  line L26 (200, 0) -> (200, 23)
  dimension "d172" = 4.6
  constraint coincident L4 L22.end
  constraint perpendicular L4 L22
  constraint coincident L2 L22.start
  constraint midpoint L2 L23.start
  constraint midpoint L4 L23.end
  constraint symmetric L22.end L23 L24.end
  constraint symmetric L22.start L23 L24.start
  constraint coincident L5.end L6.start
  constraint coincident L0.end L1.start
  constraint coincident L10.start L15.end
  constraint coincident L4 L26.end
  constraint perpendicular L4 L26
  measures "d172" distance of L3 L22
extrude "Extrude16" add sketch "Sketch5" along normal blind 3 contours L1 L2 L4 L5 L10 L25 L26 | L2 A0 A8 A12 A14 L10 L15 L24 | L4 A1 A6 L15 L24 L26 | L2 L3 L4 L11 L21 | L2 A4 A5 A13 A15 L11 L12 L20 L22 | L4 A7 A9 L12 A20 A21 A23 L20 L21 L22 bodies 31 in component "Connections"
extrude "Extrude17" add sketch "Sketch5" along normal blind 4 from surface at 3 contours L1 L2 L4 L5 L10 L25 L26 | L2 L3 L4 L11 L21 bodies 31 in component "Connections"
mirror "Mirror4" about plane through (221, -45, 7) normal (1, 0, 0) of bodies 31 30 makes body 32 at (457, 20.7677, -205.6705) makes body 33 at (451, -20.7375, -205.7333) in component "Connections"
sketch "Sketch6" plane through (455, 0, 0) normal (1, 0, 0) x (0, 0, -1) in component "Connections"
  line L0 (-14, -110) -> (0, -110)
  line L1 (0, -110) -> (0, 20)
  line L2 (0, 20) -> (-14, 20)
  line L3 (-14, 20) -> (-14, -110)
  circle A0 centre (-11.5, -55) radius 1.4
  circle A1 centre (-11.5, -45) radius 1.4
  circle A2 centre (-11.5, 15) radius 1.4
  circle A3 centre (-11.5, 5) radius 1.4
  circle A4 centre (-2.5, 5) radius 1.4
  circle A5 centre (-2.5, -15) radius 1.4
  circle A6 centre (-2.5, -5) radius 1.4
  circle A7 centre (-2.5, 15) radius 1.4
  circle A8 centre (-5, -105) radius 1.4
  circle A9 centre (-5, -95) radius 1.4
  circle A10 centre (-2.5, -55) radius 1.4
  circle A11 centre (-2.5, -45) radius 1.4
  circle A12 centre (190, 5) radius 1.4
  circle A13 centre (202.5, 15) radius 1.4
  circle A14 centre (202.5, -15) radius 1.4
  circle A15 centre (211.5, 5) radius 1.4
  circle A16 centre (211.5, 15) radius 1.4
  circle A17 centre (202.5, 5) radius 1.4
  circle A18 centre (180, 5) radius 1.4
  circle A19 centre (202.5, -5) radius 1.4
  circle A20 centre (211.5, -5) radius 1.4
  circle A21 centre (211.5, -15) radius 1.4
  line L4 (197.9, -6.1) -> (197.9, -23)
  line L5 (197.9, -23) -> (216.1, -23)
  line L6 (216.1, -23) -> (216.1, 23)
  line L7 (216.1, 23) -> (197.9, 23)
  line L8 (197.9, 23) -> (197.9, 16.1)
  line L9 (197.9, 16.1) -> (193.9, 12.1)
  line L10 (193.9, 12.1) -> (176, 12.1)
  line L11 (176, 12.1) -> (176, -2.1)
  line L12 (176, -2.1) -> (193.9, -2.1)
  line L13 (193.9, -2.1) -> (197.9, -6.1)
  line L14 (100, 10) -> (100, 0) construction
  line L15 (6.1, 12.1) -> (24, 12.1)
  circle A22 centre (-11.5, 5) radius 1.4
  circle A23 centre (10, 5) radius 1.4
  circle A24 centre (20, 5) radius 1.4
  line L16 (2.1, -6.1) -> (2.1, -23)
  line L17 (2.1, -23) -> (-16.1, -23)
  line L18 (24, -2.1) -> (6.1, -2.1)
  circle A25 centre (-2.5, -15) radius 1.4
  line L19 (24, 12.1) -> (24, -2.1)
  line L20 (6.1, -2.1) -> (2.1, -6.1)
  circle A26 centre (-2.5, -5) radius 1.4
  line L21 (-16.1, -23) -> (-16.1, 23)
  circle A27 centre (-2.5, 5) radius 1.4
  line L22 (2.1, 23) -> (2.1, 16.1)
  circle A28 centre (-2.5, 15) radius 1.4
  line L23 (2.1, 16.1) -> (6.1, 12.1)
  line L24 (-16.1, 23) -> (2.1, 23)
  circle A29 centre (-11.5, 15) radius 1.4
  line L25 (24, -0.1) -> (4.9, -0.1)
  line L26 (4.9, -0.1) -> (4.9, 10.1)
  line L27 (4.9, 10.1) -> (24, 10.1)
  circle A30 centre (10, 5) radius 1.4
  circle A31 centre (190, 5) radius 1.4
  circle A32 centre (20, 5) radius 1.4
  circle A33 centre (180, 5) radius 1.4
  arc A34 (190, 0) -> (190, 10) centre (190, 5) ccw
  line L28 (190, 10) -> (10, 10)
  arc A35 (10, 10) -> (10, 0) centre (10, 5) ccw
  line L29 (10, 0) -> (190, 0)
  line L30 (-14.1, 20.1) -> (-14.1, -110.1)
  line L31 (-14.1, -110.1) -> (0.1, -110.1)
  line L32 (0.1, -110.1) -> (0.1, 20.1)
  line L33 (0.1, 20.1) -> (-14.1, 20.1)
  dimension "d180" = 0.1
  dimension "d181" = 5.1
  dimension "d182" = 0.1
  dimension "d183" = 0.1
  dimension "d184" = 2
  constraint vertical L14
  constraint symmetric A12 L14 A23
  constraint symmetric A13 L14 A28
  constraint symmetric A14 L14 A25
  constraint symmetric A15 L14 A22
  constraint symmetric A16 L14 A29
  constraint symmetric A17 L14 A27
  constraint symmetric A18 L14 A24
  constraint symmetric A19 L14 A26
  constraint symmetric L4.start L14 L16.start
  constraint symmetric L4.end L14 L16.end
  constraint symmetric L5.end L14 L17.end
  constraint symmetric L6.end L14 L21.end
  constraint symmetric L7.end L14 L22.start
  constraint symmetric L8.end L14 L22.end
  constraint symmetric L9.end L14 L15.start
  constraint symmetric L10.end L14 L15.end
  constraint symmetric L11.end L14 L18.start
  constraint symmetric L12.end L14 L18.end
  constraint coincident L19 L25.start
  constraint perpendicular L19 L25
  constraint perpendicular L25 L26
  constraint perpendicular L19 L27
  constraint coincident L19 L27.end
  measures "d180" distance of L27 L28
  measures "d181" distance of L26 A23.centre
  measures "d182" distance of L25 L29
  measures "d184" distance of L21 L30
extrude "Extrude18" add sketch "Sketch6" along normal blind 2 separate body contours L1 L2 L3 L17 L30 L32 L33 | L1 L2 L3 L17 | L15 L16 L17 L18 L19 L20 L21 L22 L23 L24 L25 L26 L27 L30 L32 L33 | L19 L25 L26 L27 L28 A35 L29 | L19 L28 A35 L29 makes body 34 in component "Connections"
extrude "Extrude19" add sketch "Sketch6" against normal blind 2 contours L15 L16 L17 L18 L19 L20 L21 L22 L23 L24 L25 L26 L27 L30 L32 L33 bodies 34 in component "Connections"
extrude "Extrude20" add sketch "Sketch6" against normal blind 2 from surface at -2 separate body contours L15 L16 L17 L18 L19 L20 L21 L22 L23 L24 L25 L26 L27 L30 L32 L33 makes body 35 in component "Connections"
extrude "Extrude21" add sketch "Sketch6" against normal blind 2 from surface at -4 contours L1 L2 L3 L17 L30 L32 L33 | L1 L2 L3 L17 | L15 L16 L17 L18 L19 L20 L21 L22 L23 L24 L25 L26 L27 L30 L32 L33 | L19 L25 L26 L27 L28 A35 L29 | L19 L28 A35 L29 bodies 35 in component "Connections"
sketch "Sketch7" plane through (449, 0, 0) normal (-1, 0, 0) x (0, 0, 1) in component "Connections"
  line L0 (-2.1, -23) -> (16.1, -23)
  line L1 (16.1, -23) -> (16.1, 23)
  line L2 (16.1, 23) -> (-2.1, 23)
  line L3 (-2.1, 23) -> (-2.1, 16.1)
  line L4 (-2.1, 16.1) -> (-6.1, 12.1)
  line L5 (-6.1, 12.1) -> (-24, 12.1)
  line L6 (-24, 12.1) -> (-24, -2.1)
  line L7 (-24, -2.1) -> (-6.1, -2.1)
  line L8 (-6.1, -2.1) -> (-2.1, -6.1)
  line L9 (-2.1, -6.1) -> (-2.1, -23)
  circle A0 centre (2.5, 15) radius 1.4
  circle A1 centre (2.5, -15) radius 1.4
  circle A2 centre (2.5, 5) radius 1.4
  circle A3 centre (11.5, 5) radius 1.4
  circle A4 centre (-20, 5) radius 1.4
  circle A5 centre (2.5, -5) radius 1.4
  circle A6 centre (11.5, 15) radius 1.4
  circle A7 centre (-10, 5) radius 1.4
  circle A8 centre (-211.5, 5) radius 1.4
  circle A9 centre (11.5, 15) radius 1.4
  circle A10 centre (-211.5, 15) radius 1.4
  circle A11 centre (11.5, 5) radius 1.4
  arc A12 (14, 50) -> (-214, 50) centre (-100, 50) ccw
  line L10 (-214, 50) -> (-214, 0)
  line L11 (-214, 0) -> (-209, 0)
  line L12 (-209, 0) -> (-209, 50)
  arc A13 (9, 50) -> (-209, 50) centre (-100, 50) ccw
  line L13 (9, 50) -> (9, 0)
  line L14 (9, 0) -> (14, 0)
  line L15 (14, 0) -> (14, 50)
  circle A14 centre (2.5, 5) radius 1.4
  circle A15 centre (-202.5, 15) radius 1.4
  circle A16 centre (-202.5, 5) radius 1.4
  circle A17 centre (2.5, 15) radius 1.4
  line L16 (-200, 0) -> (-200, 50)
  arc A18 (0, 50) -> (-200, 50) centre (-100, 50) ccw
  line L17 (0, 50) -> (0, 0)
  line L18 (0, 0) -> (5, 0)
  line L19 (5, 0) -> (5, 50)
  arc A19 (5, 50) -> (-205, 50) centre (-100, 50) ccw
  line L20 (-205, 50) -> (-205, 0)
  line L21 (-205, 0) -> (-200, 0)
  line L22 (5, 0) -> (9, 0)
  line L23 (-2.1, 16.1) -> (-2.1, -2.5)
  line L24 (-2.1, -2.5) -> (16.1, -2.5)
  line L25 (11.5, -2.5) -> (11.5, 23)
  line L26 (7, 0) -> (7, 23) construction
  line L27 (2.5, -2.5) -> (2.5, 23)
  dimension "d195" = 2.5
  dimension "d196" = 4.6
  constraint coincident L18.end L19.start
  constraint coincident L13.end L14.start
  constraint coincident L3.end L4.start
  constraint perpendicular L22 L23
  constraint coincident L1 L24.end
  constraint perpendicular L1 L24
  constraint coincident L24 L25.start
  constraint coincident L2 L25.end
  constraint midpoint L22 L26.start
  constraint midpoint L2 L26.end
  constraint symmetric L25.start L26 L27.start
  constraint symmetric L25.end L26 L27.end
  measures "d195" distance of L22 L24
  measures "d196" distance of L1 L25
extrude "Extrude22" add sketch "Sketch7" along normal blind 3 contours L1 L2 L14 L15 L24 L25 | L14 L18 L22 L24 L25 L27 | L2 A3 A6 A9 A11 L14 L15 L25 | L2 L3 L17 L18 L23 L24 L27 | L2 A0 A2 A14 A17 L17 L18 L27 bodies 35 in component "Connections"
extrude "Extrude23" add sketch "Sketch7" against normal blind 4 from surface at 7 contours L1 L2 L14 L15 L24 L25 | L14 L18 L22 L24 L25 L27 | L2 L3 L17 L18 L23 L24 L27 bodies 35 in component "Connections"
sketch "Sketch8" plane through (0, 0, 16.1) normal (0, 0, 1) x (1, 0, 0) in component "Connections"
  line L0 (453, -23) -> (453, 23)
  line L1 (453, 23) -> (442, 23)
  line L2 (442, 23) -> (442, -2.5)
  line L3 (442, -2.5) -> (449, -2.5)
  line L4 (449, -2.5) -> (449, -23)
  line L5 (449, -23) -> (453, -23)
  line L6 (449, -2.5) -> (423, -2.5)
  line L7 (423, -2.5) -> (423, -23)
  line L8 (423, -23) -> (449, -23)
  line L9 (449, -2.5) -> (449, -23)
  circle A0 centre (431, -10) radius 1.4
  circle A1 centre (1, -10) radius 1.4
  circle A2 centre (441, -10) radius 1.4
  circle A3 centre (11, -10) radius 1.4
  arc A4 (1, -5) -> (1, -15) centre (1, -10) ccw
  line L10 (1, -15) -> (441, -15)
  arc A5 (441, -15) -> (441, -5) centre (441, -10) ccw
  line L11 (441, -5) -> (1, -5)
  line L12 (1, -15.1) -> (441, -15.1)
  arc A6 (441, -15.1) -> (441, -4.9) centre (441, -10) ccw
  line L13 (441, -4.9) -> (1, -4.9)
  arc A7 (1, -4.9) -> (1, -15.1) centre (1, -10) ccw
  line L14 (423, -17.5) -> (442, -17.5)
  line L15 (442, -17.5) -> (442, -23)
  line L16 (442, -23) -> (436.5, -17.5)
  line L17 (442, -23) -> (450.8989, -23) construction
  dimension "d205" = 8
  dimension "d214" = 2.4
  dimension "d215" = 135
  dimension "d216" = 19
  constraint coincident L3.end L4.start
  constraint perpendicular L0 L6
  constraint perpendicular L6 L7
  constraint coincident L4.end L5.start
  constraint perpendicular L7 L8
  constraint coincident L7 L14.start
  constraint perpendicular L7 L14
  constraint coincident L8 L15.end
  constraint perpendicular L8 L15
  constraint horizontal L17
  constraint coincident L14 L16.end
  constraint concentric A5 A6
  constraint concentric A4 A7
  measures "d205" distance of L7 A0.centre
  measures "d214" distance of L12 L14
  measures "d215" angle of L16 L17
  measures "d216" distance of L7 L15
extrude "Extrude24" add sketch "Sketch8" against normal blind 3.1 contours L3 L4 L6 L7 L8 L9 L12 A6 L13 L14 L15 | L14 L15 L16 | L7 L10 A5 L11 L12 A6 L13 | L7 L10 A5 L11 bodies 35 in component "Connections"
extrude "Extrude25" add sketch "Sketch8" against normal blind 4 from surface at -3.1 contours L3 L4 L6 L7 L8 L9 L12 A6 L13 L14 L15 | L14 L15 L16 bodies 35 in component "Connections"
extrude "Extrude26" add sketch "Sketch8" against normal blind 2 from surface at -7.1 contours L3 L4 L6 L7 L8 L9 L12 A6 L13 L14 L15 | L14 L15 L16 | L7 L10 A5 L11 L12 A6 L13 | L7 L10 A5 L11 bodies 35 in component "Connections"
mirror "Mirror5" about plane through (221, -45, 7) normal (1, 0, 0) of bodies 34 35 makes body 36 at (-15, -8.2386, 10.6498) makes body 37 at (-7.3333, -0.8333, 16.1) in component "Connections"
delete_body "RemoveBody1" bodies 25 in component "Along carcas"
component "Door" placed x (1, 0, 0) y (0, 1, 0) z (0, 0, 1) at (0, 0, 0)
component "Carcas" placed x (1, 0, 0) y (0, 1, 0) z (0, 0, 1) at (0, 0, 0)
component "Closing system" placed x (1, 0, 0) y (0, 1, 0) z (0, 0, 1) at (0, 0, 0)
component "Obolochka" placed x (1, 0, 0) y (0, 1, 0) z (0, 0, 1) at (0, 0, 0)
component "Along carcas" placed x (1, 0, 0) y (0, 1, 0) z (0, 0, 1) at (0, 0, 0) in component "Carcas"
component "Connections" placed x (1, 0, 0) y (0, 1, 0) z (0, 0, 1) at (0, 0, 0) in component "Carcas"
component "Transverse carcas" placed x (1, 0, 0) y (0, 1, 0) z (0, 0, 1) at (0, 0, 0) in component "Carcas"
component "High carcas" placed x (1, 0, 0) y (0, 1, 0) z (0, 0, 1) at (0, 0, 0) in component "Carcas"
equation "d121 = 450 mm - 220 mm"
named bodies: "connection for carcas", "connection for carcas (1)", "connection for carcas (2)", "connection for carcas (3)", "connection for carcas (4)", "connection for carcas (5)", "connection for carcas (6)", "connection for carcas (7)", "connection for door", "connection for door (1)"
